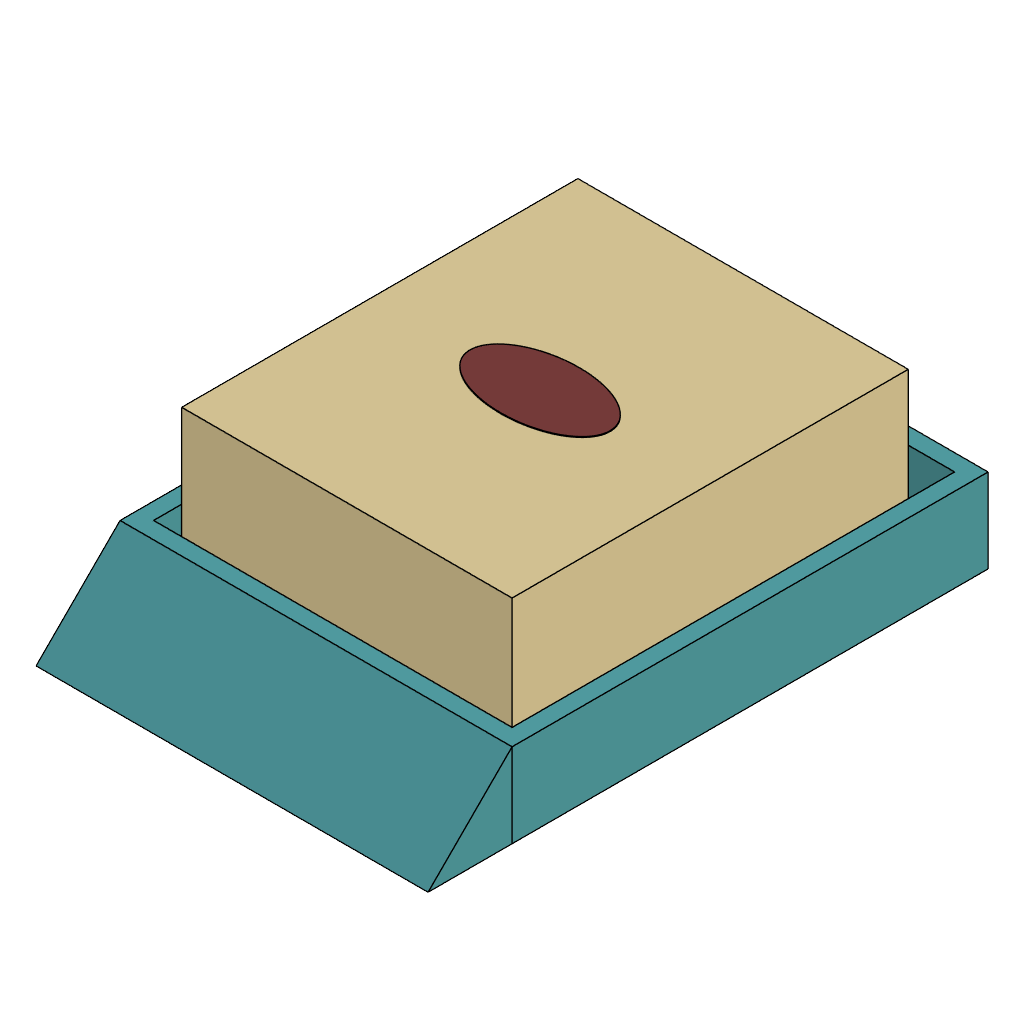
Histology-Embedded-Cassette-v01 (Autodesk Fusion 360 design; units mm, degrees)
Autodesk Fusion 360 part; units mm, degrees
sketch "Sketch1" plane through (0, 0, 0) normal (0, 0, 1) x (1, 0, 0)
  line L0 (-14, -14) -> (14, -14)
  line L1 (14, -14) -> (14, 20)
  line L2 (14, 20) -> (-14, 20)
  line L3 (-14, 20) -> (-14, -14)
extrude "Cassette plastic body" add sketch "Sketch1" along normal blind 6 makes body 1
ref_plane "WorkPlane1" through (0, 0, 6) normal (0, 0, 1) x (1, 0, 0)
sketch "Sketch2" plane through (0, 0, 6) normal (0, 0, 1) x (1, 0, 0)
  line L0 (-12.8, -12.8) -> (12.8, -12.8)
  line L1 (12.8, -12.8) -> (12.8, 18.8)
  line L2 (12.8, 18.8) -> (-12.8, 18.8)
  line L3 (-12.8, 18.8) -> (-12.8, -12.8)
extrude "Cassette cavity" cut sketch "Sketch2" against normal blind 5 bodies 1
sketch "Sketch3" plane through (0, 0, 0) normal (0, 0, 1) x (1, 0, 0)
  line L0 (-11.3, -10.8) -> (-5.5, -10.8)
  line L1 (-5.5, -10.8) -> (-5.5, -9.5)
  line L2 (-5.5, -9.5) -> (-11.3, -9.5)
  line L3 (-11.3, -9.5) -> (-11.3, -10.8)
  line L4 (-3.3, -10.8) -> (2.5, -10.8)
  line L5 (2.5, -10.8) -> (2.5, -9.5)
  line L6 (2.5, -9.5) -> (-3.3, -9.5)
  line L7 (-3.3, -9.5) -> (-3.3, -10.8)
  line L8 (4.7, -10.8) -> (10.5, -10.8)
  line L9 (10.5, -10.8) -> (10.5, -9.5)
  line L10 (10.5, -9.5) -> (4.7, -9.5)
  line L11 (4.7, -9.5) -> (4.7, -10.8)
  line L12 (-11.3, -7.3) -> (-5.5, -7.3)
  line L13 (-5.5, -7.3) -> (-5.5, -6)
  line L14 (-5.5, -6) -> (-11.3, -6)
  line L15 (-11.3, -6) -> (-11.3, -7.3)
  line L16 (-3.3, -7.3) -> (2.5, -7.3)
  line L17 (2.5, -7.3) -> (2.5, -6)
  line L18 (2.5, -6) -> (-3.3, -6)
  line L19 (-3.3, -6) -> (-3.3, -7.3)
  line L20 (4.7, -7.3) -> (10.5, -7.3)
  line L21 (10.5, -7.3) -> (10.5, -6)
  line L22 (10.5, -6) -> (4.7, -6)
  line L23 (4.7, -6) -> (4.7, -7.3)
  line L24 (-11.3, -3.8) -> (-5.5, -3.8)
  line L25 (-5.5, -3.8) -> (-5.5, -2.5)
  line L26 (-5.5, -2.5) -> (-11.3, -2.5)
  line L27 (-11.3, -2.5) -> (-11.3, -3.8)
  line L28 (-3.3, -3.8) -> (2.5, -3.8)
  line L29 (2.5, -3.8) -> (2.5, -2.5)
  line L30 (2.5, -2.5) -> (-3.3, -2.5)
  line L31 (-3.3, -2.5) -> (-3.3, -3.8)
  line L32 (4.7, -3.8) -> (10.5, -3.8)
  line L33 (10.5, -3.8) -> (10.5, -2.5)
  line L34 (10.5, -2.5) -> (4.7, -2.5)
  line L35 (4.7, -2.5) -> (4.7, -3.8)
  line L36 (-11.3, -0.3) -> (-5.5, -0.3)
  line L37 (-5.5, -0.3) -> (-5.5, 1)
  line L38 (-5.5, 1) -> (-11.3, 1)
  line L39 (-11.3, 1) -> (-11.3, -0.3)
  line L40 (-3.3, -0.3) -> (2.5, -0.3)
  line L41 (2.5, -0.3) -> (2.5, 1)
  line L42 (2.5, 1) -> (-3.3, 1)
  line L43 (-3.3, 1) -> (-3.3, -0.3)
  line L44 (4.7, -0.3) -> (10.5, -0.3)
  line L45 (10.5, -0.3) -> (10.5, 1)
  line L46 (10.5, 1) -> (4.7, 1)
  line L47 (4.7, 1) -> (4.7, -0.3)
  line L48 (-11.3, 3.2) -> (-5.5, 3.2)
  line L49 (-5.5, 3.2) -> (-5.5, 4.5)
  line L50 (-5.5, 4.5) -> (-11.3, 4.5)
  line L51 (-11.3, 4.5) -> (-11.3, 3.2)
  line L52 (-3.3, 3.2) -> (2.5, 3.2)
  line L53 (2.5, 3.2) -> (2.5, 4.5)
  line L54 (2.5, 4.5) -> (-3.3, 4.5)
  line L55 (-3.3, 4.5) -> (-3.3, 3.2)
  line L56 (4.7, 3.2) -> (10.5, 3.2)
  line L57 (10.5, 3.2) -> (10.5, 4.5)
  line L58 (10.5, 4.5) -> (4.7, 4.5)
  line L59 (4.7, 4.5) -> (4.7, 3.2)
  line L60 (-11.3, 6.7) -> (-5.5, 6.7)
  line L61 (-5.5, 6.7) -> (-5.5, 8)
  line L62 (-5.5, 8) -> (-11.3, 8)
  line L63 (-11.3, 8) -> (-11.3, 6.7)
  line L64 (-3.3, 6.7) -> (2.5, 6.7)
  line L65 (2.5, 6.7) -> (2.5, 8)
  line L66 (2.5, 8) -> (-3.3, 8)
  line L67 (-3.3, 8) -> (-3.3, 6.7)
  line L68 (4.7, 6.7) -> (10.5, 6.7)
  line L69 (10.5, 6.7) -> (10.5, 8)
  line L70 (10.5, 8) -> (4.7, 8)
  line L71 (4.7, 8) -> (4.7, 6.7)
  line L72 (-11.3, 10.2) -> (-5.5, 10.2)
  line L73 (-5.5, 10.2) -> (-5.5, 11.5)
  line L74 (-5.5, 11.5) -> (-11.3, 11.5)
  line L75 (-11.3, 11.5) -> (-11.3, 10.2)
  line L76 (-3.3, 10.2) -> (2.5, 10.2)
  line L77 (2.5, 10.2) -> (2.5, 11.5)
  line L78 (2.5, 11.5) -> (-3.3, 11.5)
  line L79 (-3.3, 11.5) -> (-3.3, 10.2)
  line L80 (4.7, 10.2) -> (10.5, 10.2)
  line L81 (10.5, 10.2) -> (10.5, 11.5)
  line L82 (10.5, 11.5) -> (4.7, 11.5)
  line L83 (4.7, 11.5) -> (4.7, 10.2)
  line L84 (-11.3, 13.7) -> (-5.5, 13.7)
  line L85 (-5.5, 13.7) -> (-5.5, 15)
  line L86 (-5.5, 15) -> (-11.3, 15)
  line L87 (-11.3, 15) -> (-11.3, 13.7)
  line L88 (-3.3, 13.7) -> (2.5, 13.7)
  line L89 (2.5, 13.7) -> (2.5, 15)
  line L90 (2.5, 15) -> (-3.3, 15)
  line L91 (-3.3, 15) -> (-3.3, 13.7)
  line L92 (4.7, 13.7) -> (10.5, 13.7)
  line L93 (10.5, 13.7) -> (10.5, 15)
  line L94 (10.5, 15) -> (4.7, 15)
  line L95 (4.7, 15) -> (4.7, 13.7)
extrude "24 drainage slots" cut sketch "Sketch3" along normal blind 1.1 bodies 1
ref_plane "WorkPlane2" through (-14, 0, 0) normal (1, 0, 0) x (0, 1, 0)
sketch "Sketch4" plane through (-14, 0, 0) normal (1, 0, 0) x (0, 0, -1)
  line L0 (0, -20) -> (0, -14)
  line L1 (0, -14) -> (-6, -14)
  line L2 (-6, -14) -> (0, -20)
extrude "45 degree labeling face" add sketch "Sketch4" along normal blind 28 separate body makes body 2
ref_plane "WorkPlane3" through (0, 0, 5) normal (0, 0, 1) x (1, 0, 0)
sketch "Sketch5" plane through (0, 0, 5) normal (0, 0, 1) x (1, 0, 0)
  line L0 (-11.8, -11.8) -> (11.8, -11.8)
  line L1 (11.8, -11.8) -> (11.8, 16.5)
  line L2 (11.8, 16.5) -> (-11.8, 16.5)
  line L3 (-11.8, 16.5) -> (-11.8, -11.8)
extrude "Paraffin embedded block" add sketch "Sketch5" along normal blind 8 separate body makes body 3
ref_plane "WorkPlane4" through (0, 0, 13) normal (0, 0, 1) x (1, 0, 0)
sketch "Sketch6" plane through (0, 0, 13) normal (0, 0, 1) x (1, 0, 0)
  ellipse E0 centre (0, 2) end of major axis (5, 2) minor radius 2.8
  line L0 (-5, 2) -> (5, 2) construction
  line L1 (0, 4.8) -> (0, -0.8) construction
  constraint coincident E0 L0.start
  constraint coincident E0 L0.end
  constraint coincident E0 L1.start
  constraint coincident E0 L1.end
extrude "Tissue at sectioning face - schematic" add sketch "Sketch6" along normal blind 0.05 separate body makes body 4
equation "cassetteWidth = 28 mm" comment "Generic cassette prototype; measure target consumable before fit testing"
equation "cassetteLength = 40 mm" comment "Generic cassette prototype; measure target consumable before fit testing"
equation "cassetteHeight = 6 mm" comment "Generic cassette prototype; measure target consumable before fit testing"
equation "waxHeight = 8 mm" comment "Generic cassette prototype; measure target consumable before fit testing"
equation "d5 = cassetteHeight"
equation "d15 = cassetteWidth"
equation "d19 = waxHeight"
named bodies: "24 drainage slots", "45 degree labeling face", "Paraffin embedded block", "Tissue at sectioning face - schematic"
